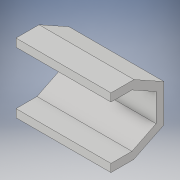
# Autodesk Inventor part: BatteryHolder
Saved by Autodesk Inventor 2018 (Build 220112000, 112)
## iProperties
Created: 2018-11-16
Part Number: BatteryHolder
Material: Generic
Document SubType Name: Modeling
Designer: iki
Density: 1 g/cm^3
Appearance: Default
Author: iki
Autodesk Inventor part; units mm, degrees
ref_plane "YZ Plane" through (0, 0, 0) normal (1, 0, 0) x (0, 1, 0)
ref_plane "XZ Plane" through (0, 0, 0) normal (0, 1, 0) x (-1, 0, 0)
ref_plane "XY Plane" through (0, 0, 0) normal (0, 0, 1) x (1, 0, 0)
sketch "Sketch1" plane through (0, 0, 0) normal (1, 0, 0) x (0, 1, 0)
  line L0 (25346.4946, 38060.2067) -> (25328.8946, 38060.2067)
  line L1 (0, -1) -> (0, -18.6)
  line L2 (-15.25, -26.1) -> (-28.5, -26.1)
  line L3 (-15.25, 7.5) -> (-28.5, 7.5)
  line L4 (-15.25, 7.5) -> (0, -1)
  line L5 (0, -18.6) -> (-15.25, -26.1)
  line L6 (-28.5, 12.5) -> (-13.9507, 12.5)
  line L7 (-13.9507, 12.5) -> (5, 1.9373)
  line L8 (5, 1.9373) -> (5, -21.7129)
  line L9 (5, -21.7129) -> (-14.087, -31.1)
  line L10 (-14.087, -31.1) -> (-28.5, -31.1)
  line L11 (-28.5, 12.5) -> (-28.5, 7.5)
  line L12 (-28.5, -26.1) -> (-28.5, -31.1)
  dimension "d2" = 17.6
  dimension "d8" = 5
  constraints: 26 end point, 2 vertical, 1 collinear, 1 horizontal, 4 other
  measures "d2" distance of L1.start L1.end
  measures "d8" distance between parallel lines of L3 L6
extrude "Extrusion1" add sketch "Sketch1" along normal blind 60
body "Solid1"
